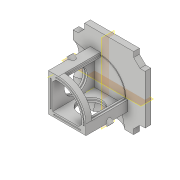
# Autodesk Inventor part: 20_Cube_Insert_Lightsheet_FEPTube_Flowcube_v3
Saved by Autodesk Inventor 2022 (Build 260153000, 153)
## iProperties
Created: 2019-07-01
Part Number: 20_Cube_Insert_Lightsheet_FEPTube_Flowcube_v3
Material: Generic
Document SubType Name: Modeling
Designer: diederichbenedict
Density: 1 g/cm^3
Appearance: Default
Author: diederichbenedict
Autodesk Inventor part; units mm, degrees
ref_plane "YZ Plane" through (0, 0, 0) normal (1, 0, 0) x (0, 1, 0)
ref_plane "XZ Plane" through (0, 0, 0) normal (0, 1, 0) x (-1, 0, 0)
ref_plane "Work Plane1" through (0, 0, 10) normal (0, 0, 1) x (1, 0, 0)
sketch "Sketch1" plane through (0, 0, 10) normal (0, 0, 1) x (1, 0, 0)
  line L0 (-4.0299, -0.3538) -> (-2.2322, 1.4439) construction
  arc A0 (-1.4439, 2.2322) -> (-2.2322, 1.4439) centre (-0.9299, 0.9299) ccw construction
  line L1 (-1.4439, 2.2322) -> (0.3538, 4.0299) construction
  line L2 (-37.8299, 42.8299) -> (-37.8299, 37.8299) construction
  line L3 (-37.8299, 37.8299) -> (-42.9208, 37.8299) construction
  line L4 (-37.8299, 42.2137) -> (-37.8299, 45.8299) construction
  line L5 (-37.8299, 45.8299) -> (-4.0299, 45.8299) construction
  line L6 (-4.0299, 45.8299) -> (-4.0299, 42.2137) construction
  line L7 (-4.0299, 4.0299) -> (0.3538, 4.0299) projected
  circle A1 centre (-20.9299, 20.9299) radius 17.5 projected
  line L8 (-20.9299, 58.9723) -> (17.1124, 20.9299) construction
  line L9 (17.1124, 20.9299) -> (-20.9299, -17.1124) construction
  line L10 (-20.9299, -17.1124) -> (-58.9723, 20.9299) construction
  line L11 (-58.9723, 20.9299) -> (-20.9299, 58.9723) construction
  line L12 (-20.9299, 58.9723) -> (-20.9299, -17.1124) construction
  line L13 (17.1124, 20.9299) -> (-58.9723, 20.9299) construction
  line L14 (-20.9299, 58.9723) -> (32.8701, 58.9723) construction
  line L15 (-43.4299, 43.4299) -> (1.5701, 43.4299) construction
  line L16 (1.5701, 43.4299) -> (1.5701, -1.5701) construction
  line L17 (1.5701, -1.5701) -> (-43.4299, -1.5701) construction
  line L18 (-43.4299, -1.5701) -> (-43.4299, 43.4299) construction
  line L19 (-43.4299, 43.4299) -> (1.5701, -1.5701) construction
  line L20 (1.5701, 43.4299) -> (-43.4299, -1.5701) construction
  line L21 (-43.4299, 5.3876) -> (-43.4299, 36.4723)
  line L22 (-43.4299, 36.4723) -> (-36.4723, 43.4299)
  line L23 (-36.4723, 43.4299) -> (-5.3876, 43.4299)
  line L24 (-5.3876, 43.4299) -> (1.5701, 36.4723)
  line L25 (1.5701, 36.4723) -> (1.5701, 5.3876)
  line L26 (1.5701, 5.3876) -> (-5.3876, -1.5701)
  line L27 (-5.3876, -1.5701) -> (-36.4723, -1.5701)
  line L28 (-36.4723, -1.5701) -> (-43.4299, 5.3876)
  line L29 (-4.0299, 42.2137) -> (-37.8299, 42.2137) projected
  line L30 (-4.0299, -0.3538) -> (-4.0299, 4.0299) projected
  circle A2 centre (-20.9299, 20.9299) radius 1.5
  line L31 (-10.9299, 10.9299) -> (-30.9299, 10.9299) construction
  line L32 (-30.9299, 10.9299) -> (-30.9299, 30.9299) construction
  line L33 (-30.9299, 30.9299) -> (-10.9299, 30.9299) construction
  line L34 (-10.9299, 30.9299) -> (-10.9299, 10.9299) construction
  line L35 (-10.9299, 10.9299) -> (-30.9299, 30.9299) construction
  line L36 (-30.9299, 10.9299) -> (-10.9299, 30.9299) construction
  circle A3 centre (-30.9299, 30.9299) radius 1.4
  circle A4 centre (-30.9299, 10.9299) radius 1.4
  circle A5 centre (-10.9299, 10.9299) radius 1.4
  line L37 (-45.8299, 37.8299) -> (-42.0723, 37.8299) construction
  line L38 (-42.1723, 37.7299) -> (-45.8299, 37.7299)
  line L39 (-45.8299, 37.7299) -> (-45.8299, 4.1299)
  line L40 (-45.8299, 4.1299) -> (-42.1723, 4.1299)
  line L41 (-42.1723, 4.1299) -> (-42.1723, 37.7299)
  line L42 (-45.8299, 4.0299) -> (-42.0723, 4.0299) construction
  line L43 (-45.8299, 37.8299) -> (-42.0723, 37.8299) projected
  line L44 (-37.7299, 45.8299) -> (-4.1299, 45.8299)
  line L45 (-4.1299, 45.8299) -> (-4.1299, 42.1723)
  line L46 (-4.1299, 42.1723) -> (-37.7299, 42.1723)
  line L47 (-37.7299, 42.1723) -> (-37.7299, 45.8299)
  line L48 (0.4701, 37.8299) -> (0.4701, 4.0299) construction
  line L49 (0.4701, 4.0299) -> (3.9701, 4.0299) construction
  line L50 (3.9701, 37.8299) -> (3.9701, 4.0299) construction
  line L51 (0.4701, 37.8299) -> (3.9701, 37.8299) construction
  line L52 (-45.8299, -3.9701) -> (-4.0299, -3.9701) construction
  line L53 (0.3124, 37.7299) -> (3.9701, 37.7299)
  line L54 (3.9701, 37.7299) -> (3.9701, 4.1299)
  line L55 (3.9701, 4.1299) -> (0.3124, 4.1299)
  line L56 (0.3124, 4.1299) -> (0.3124, 37.7299)
  line L57 (-4.1713, -0.3538) -> (-37.7299, -0.3538)
  line L58 (-37.7299, -0.3538) -> (-37.7299, -3.9701)
  line L59 (-37.7299, -3.9701) -> (-4.1713, -3.9701)
  line L60 (-4.1713, -3.9701) -> (-4.1713, -0.3538)
  point P0 (-37.8299, 4.0299)
  dimension "d18" = 53.8
  dimension "d19" = 45
  dimension "d20" = 53.8
  dimension "d21" = 45
  dimension "d22" = 45
  dimension "d30" = 20
  dimension "d31" = 20
  dimension "d32" = 2.8
  dimension "d33" = 2.8
  dimension "d34" = 2.8
  dimension "d35" = 3
  dimension "d36" = 0.1
  dimension "d37" = 0.1
  dimension "d38" = 0.1
  dimension "d39" = 0.1
  constraints: 86 end point, 21 point on line, 14 parallel, 8 perpendicular, 7 horizontal, 7 midpoint, 4 centre point, 4 coincident, 1 equal length
  measures "d18" distance of L8.start L8.end
  measures "d19" angle of L8 L14
  measures "d20" distance of L8.end L9.end
  measures "d21" distance of L16.end L17.end
  measures "d22" distance of L15.end L16.end
  measures "d30" distance of L32.end L33.end
  measures "d31" distance of L31.end L32.end
  measures "d32" diameter of A3
  measures "d33" diameter of A4
  measures "d34" diameter of A5
  measures "d35" diameter of A2
  measures "d36" distance between parallel lines of L38 L43
  measures "d37" distance between parallel lines of L40 L42
  measures "d38" distance between parallel lines of L45 L6
  measures "d39" distance between parallel lines of L4 L47
extrude "Extrusion1" add sketch "Sketch1" along normal blind 3 contours L30 L26 L57 L28 L41 L22 L46 L24 L56 L7 | L7 L26 L30 | L56 L24 L25 L26 | L26 L25 L24 L53 L54 L55 | L60 L59 L58 L57 L28 L27 L26 | L26 L27 L28 L57 | L46 L22 L29 L24 | L24 L29 L45 | L40 L39 L38 L22 L21 L28 | L28 L21 L22 L41 | L29 L22 L23 L24 | L24 L23 L22 L29 L47 L44 L45 | L47 L29 L22 | A1 | A2 | A3 | A4 | A5
sketch "Skizze4" plane through (0, 0, 13) normal (0, 0, 1) x (1, 0, 0)
  line L0 (-37.7299, 42.1723) -> (-42.1723, 37.7299) projected
  line L1 (-42.1723, 37.7299) -> (-45.8299, 37.7299) projected
  line L2 (-45.8299, 37.7299) -> (-45.8299, 4.1299) construction
  line L3 (-45.8299, 4.1299) -> (-42.1723, 4.1299) projected
  line L4 (-42.1723, 4.1299) -> (-37.6885, -0.3538) projected
  line L5 (-37.6885, -0.3538) -> (-37.7299, -0.3538) projected
  line L6 (-37.7299, -0.3538) -> (-37.7299, -3.9701) projected
  line L7 (-37.7299, -3.9701) -> (-4.1713, -3.9701) construction
  line L8 (-4.1713, -3.9701) -> (-4.1713, -0.3538) projected
  line L9 (-4.1713, -0.3538) -> (0.3124, 4.1299) projected
  line L10 (0.3124, 4.1299) -> (3.9701, 4.1299) projected
  line L11 (3.9701, 4.1299) -> (3.9701, 37.7299) construction
  line L12 (3.9701, 37.7299) -> (0.3124, 37.7299) projected
  line L13 (0.3124, 37.7299) -> (-4.1299, 42.1723) projected
  line L14 (-4.1299, 42.1723) -> (-4.1299, 45.8299) projected
  line L15 (-4.1299, 45.8299) -> (-37.7299, 45.8299) construction
  line L16 (-37.7299, 45.8299) -> (-37.7299, 42.1723) projected
  line L17 (-37.9299, 46.0299) -> (-3.9299, 46.0299) construction
  line L18 (-3.9299, 46.0299) -> (-3.9299, 42.2551)
  line L19 (-3.9299, 42.2551) -> (0.3953, 37.9299)
  line L20 (0.3953, 37.9299) -> (4.1701, 37.9299)
  line L21 (4.1701, 37.9299) -> (4.1701, 3.9299) construction
  line L22 (4.1701, 3.9299) -> (0.3953, 3.9299)
  line L23 (0.3953, 3.9299) -> (-3.9713, -0.4367)
  line L24 (-3.9713, -0.4367) -> (-3.9713, -4.1701)
  line L25 (-3.9713, -4.1701) -> (-37.9299, -4.1701) construction
  line L26 (-37.9299, -4.1701) -> (-37.9299, -0.3953)
  line L27 (-37.9299, -0.3953) -> (-42.2551, 3.9299)
  line L28 (-42.2551, 3.9299) -> (-46.0299, 3.9299)
  line L29 (-46.0299, 3.9299) -> (-46.0299, 37.9299) construction
  line L30 (-46.0299, 37.9299) -> (-42.2551, 37.9299)
  line L31 (-42.2551, 37.9299) -> (-37.9299, 42.2551)
  line L32 (-37.9299, 42.2551) -> (-37.9299, 46.0299)
  line L33 (-45.8299, 37.7299) -> (-45.8299, 37.9299)
  line L34 (-4.1299, 45.8299) -> (-37.7299, 45.8299) projected
  line L35 (-37.7299, 45.8299) -> (-37.9299, 45.8299)
  line L36 (-4.1299, 45.8299) -> (-3.9299, 45.8299)
  line L37 (3.9701, 37.7299) -> (3.9701, 37.9299)
  line L38 (3.9701, 4.1299) -> (3.9701, 37.7299) projected
  line L39 (3.9701, 4.1299) -> (3.9701, 3.9299)
  line L40 (-4.1713, -3.9701) -> (-3.9713, -3.9701)
  line L41 (-37.7299, -3.9701) -> (-37.9299, -3.9701)
  line L42 (-45.8299, 4.1299) -> (-45.8299, 3.9299)
  point P0 (0, 0)
  dimension "d40" = 0.2
  constraints: 48 end point, 12 point on line, 4 perpendicular, 15 other
  measures "d40" distance between parallel lines of L15 L17
extrude "IM_offset" add sketch "Skizze4" against normal up to surface (3 mm away)
ref_plane "Arbeitsebene5" through (-20.9299, 3.9299, 10) normal (1, 0, 0) x (0, 0, -1)
ref_plane "Arbeitsebene6" through (-37.9299, 20.9299, 10) normal (0, 1, 0) x (1, 0, 0)
sketch "Skizze25" plane through (0, 0, 13) normal (0, 0, 1) x (1, 0, 0)
  line L0 (3.9701, 3.9299) -> (3.9701, 37.9299) projected
  line L1 (3.9701, 37.9299) -> (0.3953, 37.9299) projected
  line L2 (0.3953, 37.9299) -> (-3.9299, 42.2551) projected
  line L3 (-3.9299, 42.2551) -> (-3.9299, 45.8299) projected
  line L4 (-3.9299, 45.8299) -> (-37.9299, 45.8299) projected
  line L5 (-37.9299, 45.8299) -> (-37.9299, 42.2551) projected
  line L6 (-37.9299, 42.2551) -> (-42.2551, 37.9299) projected
  line L7 (-42.2551, 37.9299) -> (-45.8299, 37.9299) projected
  line L8 (-45.8299, 37.9299) -> (-45.8299, 3.9299) projected
  line L9 (-42.2551, 3.9299) -> (-45.8299, 3.9299) projected
  line L10 (-37.9299, -0.3953) -> (-42.2551, 3.9299) projected
  line L11 (-37.9299, -3.9701) -> (-37.9299, -0.3953) projected
  line L12 (-3.9713, -3.9701) -> (-37.9299, -3.9701) projected
  line L13 (-3.9713, -3.9701) -> (-3.9713, -0.4367) projected
  line L14 (-3.9713, -0.4367) -> (0.3953, 3.9299) projected
  line L15 (0.3953, 3.9299) -> (3.9701, 3.9299) projected
  line L16 (-9.2627, 11.384) -> (-30.4759, 32.5972)
  line L17 (-11.384, 9.2627) -> (-32.5972, 30.4759)
  line L18 (-10.9506, 30.9092) -> (-30.9506, 30.9092)
  line L19 (-30.9506, 30.9092) -> (-30.9506, 10.9092)
  line L20 (-30.9506, 10.9092) -> (-10.9506, 10.9092)
  line L21 (-10.9506, 10.9092) -> (-10.9506, 30.9092)
  line L22 (-10.9506, 30.9092) -> (-30.9506, 10.9092) construction
  line L23 (-30.9506, 30.9092) -> (-10.9506, 10.9092) construction
  line L24 (-7.9506, 33.9092) -> (-33.9506, 33.9092)
  line L25 (-33.9506, 33.9092) -> (-33.9506, 7.9092)
  line L26 (-33.9506, 7.9092) -> (-7.9506, 7.9092)
  line L27 (-7.9506, 7.9092) -> (-7.9506, 33.9092)
  line L28 (-10.9506, 14.9092) -> (-7.9506, 14.9092)
  line L29 (-26.9506, 30.9092) -> (-26.9506, 33.9092)
  line L30 (-13.0305, 10.9092) -> (-10.9506, 13.072)
  line L31 (-30.9506, 28.8293) -> (-28.7879, 30.9092)
  point P0 (0, 0)
  point P1 (-20.9506, 20.9092)
  dimension "d150" = 20
  dimension "d151" = 20
  dimension "d152" = 3
  dimension "d153" = 7
  dimension "d154" = 7
  constraints: 32 end point, 12 point on line, 4 parallel, 3 perpendicular, 2 horizontal, 2 midpoint, 9 other
  measures "d150" distance of L20.end L19.end
  measures "d151" distance of L19.end L18.end
  measures "d152" distance between parallel lines of L21 L27
  measures "d153" distance between parallel lines of L25 L29
  measures "d154" distance between parallel lines of L26 L28
extrude "Extrusion21" add sketch "Skizze25" along normal blind 25 contours L21 L28 L27 L26 L25 L24 L29 L18 L19 L20 | L21 L20 L30 | L31 L19 L18
sketch "Skizze26" plane through (0, 0, 38) normal (0, 0, 1) x (1, 0, 0)
  line L0 (-7.9506, 7.9092) -> (-7.9506, 14.9092) projected
  line L1 (-7.9506, 14.9092) -> (-10.9506, 14.9092) projected
  line L2 (-10.9506, 14.9092) -> (-10.9506, 13.072) projected
  line L3 (-13.0305, 10.9092) -> (-30.9506, 10.9092) projected
  line L4 (-30.9506, 10.9092) -> (-30.9506, 28.8293) projected
  line L5 (-28.7879, 30.9092) -> (-26.9506, 30.9092) projected
  line L6 (-26.9506, 30.9092) -> (-26.9506, 33.9092) projected
  line L7 (-26.9506, 33.9092) -> (-33.9506, 33.9092) projected
  line L8 (-33.9506, 33.9092) -> (-33.9506, 7.9092) projected
  line L9 (-33.9506, 7.9092) -> (-7.9506, 7.9092) projected
  arc A0 (-10.9506, 14.9092) -> (-26.9506, 30.9092) centre (-26.9506, 14.9092) ccw
  line L10 (-10.9506, 14.9092) -> (-7.9506, 14.9092) projected
  arc A1 (-7.9506, 14.9092) -> (-26.9506, 33.9092) centre (-26.9506, 14.9092) ccw
  line L11 (-10.9506, 13.072) -> (-13.0305, 10.9092) projected
  line L12 (-30.9506, 28.8293) -> (-28.7879, 30.9092) projected
  point P0 (0, 0)
  constraints: 4 point on circle, 3 tangent, 2 centre point
extrude "Extrusion22" add sketch "Skizze26" along normal blind 4 contours L9 L8 L7 L6 L5 L12 L4 L3 L11 L2 L1 L0 | L1 A0 L6 A1
sketch "Skizze27" plane through (0, 0, 42) normal (0, 0, 1) x (1, 0, 0)
  line L0 (-26.9506, 33.9092) -> (-33.9506, 33.9092) projected
  line L1 (-33.9506, 33.9092) -> (-33.9506, 7.9092) projected
  line L2 (-33.9506, 7.9092) -> (-7.9506, 7.9092) projected
  line L3 (-7.9506, 7.9092) -> (-7.9506, 14.9092) projected
  arc A0 (-7.9506, 14.9092) -> (-26.9506, 33.9092) centre (-26.9506, 14.9092) ccw projected
  line L4 (-26.9506, 32.6592) -> (-32.7006, 32.6592)
  line L5 (-32.7006, 32.6592) -> (-32.7006, 9.1592)
  line L6 (-32.7006, 9.1592) -> (-9.2006, 9.1592)
  line L7 (-9.2006, 9.1592) -> (-9.2006, 14.9092)
  arc A1 (-9.2006, 14.9092) -> (-26.9506, 32.6592) centre (-26.9506, 14.9092) ccw
  line L8 (-26.9506, 32.0592) -> (-32.1006, 32.0592)
  line L9 (-32.1006, 32.0592) -> (-32.1006, 9.7592)
  line L10 (-32.1006, 9.7592) -> (-9.8006, 9.7592)
  line L11 (-9.8006, 9.7592) -> (-9.8006, 14.9092)
  arc A2 (-9.8006, 14.9092) -> (-26.9506, 32.0592) centre (-26.9506, 14.9092) ccw
  line L12 (-9.2006, 13.072) -> (-9.8006, 13.072)
  line L13 (-28.7879, 32.0592) -> (-28.7879, 32.6592)
  line L14 (-30.2006, 9.1592) -> (-11.7006, 9.1592)
  line L15 (-11.7006, 9.1592) -> (-11.7006, 9.7592)
  line L16 (-11.7006, 9.7592) -> (-30.2006, 9.7592)
  line L17 (-30.2006, 9.7592) -> (-30.2006, 9.1592)
  line L18 (-30.2006, 9.1592) -> (-11.7006, 9.7592) construction
  line L19 (-11.7006, 9.1592) -> (-30.2006, 9.7592) construction
  line L20 (-32.7006, 30.1592) -> (-32.1006, 30.1592)
  line L21 (-32.1006, 30.1592) -> (-32.1006, 11.6592)
  line L22 (-32.1006, 11.6592) -> (-32.7006, 11.6592)
  line L23 (-32.7006, 11.6592) -> (-32.7006, 30.1592)
  line L24 (-32.7006, 30.1592) -> (-32.1006, 11.6592) construction
  line L25 (-32.1006, 30.1592) -> (-32.7006, 11.6592) construction
  point P0 (0, 0)
  point P1 (-20.9506, 9.4592)
  point P2 (-20.9506, 9.1592)
  point P3 (-32.4006, 20.9092)
  point P4 (-32.7006, 20.9092)
  point P5 (-28.7879, 30.9092)
  point P6 (-10.9506, 13.072)
  dimension "d159" = 0.6
  dimension "d160" = 1.25
  dimension "d163" = 18.5
  dimension "d164" = 18.5
  dimension "d173" = 0
  dimension "d174" = 0
  constraints: 44 end point, 8 midpoint, 6 point on line, 4 parallel, 4 perpendicular, 4 point on circle, 2 centre point, 2 horizontal, 4 other
  measures "d159" radial gap between concentric circles of A2 A1
  measures "d160" distance between parallel lines of L7 L3
  measures "d163" distance of L16.end L15.end
  measures "d164" distance of L20.end L21.end
  measures "d173" vertical distance of L12.end point (-10.951, 13.072)
  measures "d174" distance from line of point (-28.788, 30.909) L13
extrude "Extrusion23" cut sketch "Skizze27" against normal blind 30 contours A1 L7 L12 L11 A2 L8 L13 L4 | L20 L9 L22 L5 | L6 L17 L10 L15
sketch "Skizze28" plane through (-33.9506, 7.9092, 13) normal (-1, 0, 0) x (0, 0, 1)
  line L0 (51.2, 13.0207) -> (-25.1, 13.0207)
  circle A0 centre (13.05, 13.0207) radius 8
  point P0 (-13, -7.9092)
  dimension "d165" = 16
  constraints: 2 end point, 1 centre point, 1 horizontal, 1 midpoint, 2 other
  measures "d165" diameter of A0
extrude "Extrusion24" cut sketch "Skizze28" against normal blind 4
sketch "Skizze29" plane through (-33.9506, 7.9092, 13) normal (0, -1, 0) x (1, 0, 0)
  line L0 (0, 5.05) -> (0, 21.05) projected
  circle A0 centre (13.0499, 13.05) radius 8
  point P0 (33.9506, -13)
  dimension "d168" = 16
  constraints: 1 centre point
  measures "d168" diameter of A0
extrude "Extrusion25" cut sketch "Skizze29" against normal blind 4
ref_plane "Arbeitsebene7" through (-20.9299, 20.9299, 26.13) normal (-0.7071068, 0.7071068, 0) x (0.7071068, 0.7071068, 0)
sketch "Skizze30" plane through (-20.9299, 20.9299, 26.13) normal (-0.7071068, 0.7071068, 0) x (0.7071068, 0.7071068, 0)
  circle A0 centre (0, 0) radius 1.2 projected
  point P0 (0, 26.13)
extrude "Extrusion26" cut sketch "Skizze30" along normal through all both and the other way through all
ref_plane "Arbeitsebene8" through (-30.8674, 33.0715, 13) normal (0.6931675, -0.7207765, 0) x (0.7207765, 0.6931675, 0)
sketch "Skizze31" plane through (-30.8674, 33.0715, 13) normal (0.6931675, -0.7207765, 0) x (0.7207765, 0.6931675, 0)
  ellipse E0 centre (-1.5463, 13.13) end of major axis (-1.5463, 14.63) minor radius 1.4997 projected
  ellipse E1 centre (-1.5463, 13.13) end of major axis (-1.5463, 14.33) minor radius 1.1998 projected
  circle A0 centre (-1.5463, 13.13) radius 2
  point P0 (-0.6756, -13)
  dimension "d176" = 4
  constraints: 1 centre point, 1 coincident, 2 other
  measures "d176" diameter of A0
extrude "Extrusion27" add sketch "Skizze31" against normal blind 4 contours E0 | A0
sketch "Skizze32" plane through (0, 0, 10) normal (0, 0, -1) x (-1, 0, 0)
  line L0 (3.9713, -3.9701) -> (37.9299, -3.9701) projected
  line L1 (37.9299, -3.9701) -> (37.9299, -0.3953) projected
  line L2 (37.9299, -0.3953) -> (42.2551, 3.9299) projected
  line L3 (42.2551, 3.9299) -> (45.8299, 3.9299) projected
  line L4 (45.8299, 3.9299) -> (45.8299, 37.9299) projected
  line L5 (45.8299, 37.9299) -> (42.2551, 37.9299) projected
  line L6 (42.2551, 37.9299) -> (37.9299, 42.2551) projected
  line L7 (37.9299, 42.2551) -> (37.9299, 45.8299) projected
  line L8 (37.9299, 45.8299) -> (3.9299, 45.8299) projected
  line L9 (3.9299, 45.8299) -> (3.9299, 42.2551) projected
  line L10 (3.9299, 42.2551) -> (-0.3953, 37.9299) projected
  line L11 (-0.3953, 37.9299) -> (-3.9701, 37.9299) projected
  line L12 (-3.9701, 37.9299) -> (-3.9701, 3.9299) projected
  line L13 (-3.9701, 3.9299) -> (-0.3953, 3.9299) projected
  line L14 (-0.3953, 3.9299) -> (3.9713, -0.4367) projected
  line L15 (3.9713, -0.4367) -> (3.9713, -3.9701) projected
  point P0 (0, 0)
extrude "Extrusion28" add sketch "Skizze32" along normal blind 1
sketch "Skizze33" plane through (-37.9299, -3.9701, 13) normal (0, -1, 0) x (1, 0, 0)
  circle A0 centre (17.0292, 13.05) radius 8 projected
  circle A1 centre (17.0292, 13.05) radius 17.05
  line L0 (33.9586, -4) -> (0, -4) projected
  line L1 (33.9586, 11.0253) -> (0, 11.0253)
  line L2 (33.9586, 11.0253) -> (67.9172, 11.0253) construction
  point P0 (37.9299, -13)
  point P1 (0.0999, 11.0253)
  dimension "d183" = 180
  constraints: 4 end point, 2 horizontal, 1 coincident, 1 collinear, 3 other
  measures "d183" angle of L1 L2
extrude "Extrusion29" cut sketch "Skizze33" against normal up to surface (11.8793 mm away) draft -8 contours L1 A0 | A0 L1 A1 picked at (14.6826, 10.4336) picked at (30.5692, 9.6928)
mirror "Spiegeln2" about plane through (-20.9299, 20.9299, 26.13) normal (-0.7071068, 0.7071068, 0) of "Extrusion27", "Extrusion29"
body "Solid1"
